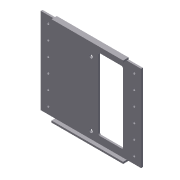
# Autodesk Inventor part: DriveTrain_MotorMount
Saved by Autodesk Inventor 2012 (Build 160160000, 160)
## iProperties
Created: 2012-01-08
Part Number: DriveTrain_MotorMount
Material: Aluminum-6061
Document SubType Name: Modeling
Designer: JesseK
Density: 2.71 g/cm^3
Mass: 222.88 g
Surface Area: 561.797 cm^2
Volume: 82.2435 cm^3
Author: JesseK
Autodesk Inventor part; units mm, degrees
ref_plane "YZ Plane" through (0, 0, 0) normal (1, 0, 0) x (0, 1, 0)
ref_plane "XZ Plane" through (0, 0, 0) normal (0, 1, 0) x (-1, 0, 0)
ref_plane "XY Plane" through (0, 0, 0) normal (0, 0, 1) x (1, 0, 0)
sketch "Sketch1" plane through (0, 0, 0) normal (0, 0, 1) x (1, 0, 0)
  line L0 (177.8, 0) -> (177.8, 152.4)
  line L1 (0, 152.4) -> (0, 0)
  line L2 (152.4, 152.4) -> (152.4, 155.575)
  line L3 (152.4, 155.575) -> (25.4, 155.575)
  line L4 (25.4, 155.575) -> (25.4, 152.4)
  line L5 (0, 152.4) -> (25.4, 152.4)
  line L6 (152.4, 152.4) -> (177.8, 152.4)
  line L7 (152.4, 0) -> (152.4, -3.175)
  line L8 (152.4, -3.175) -> (25.4, -3.175)
  line L9 (25.4, -3.175) -> (25.4, 0)
  line L10 (0, 0) -> (25.4, 0)
  line L11 (152.4, 0) -> (177.8, 0)
  dimension "d0" = 152.4
  dimension "d1" = 177.8
  dimension "d18" = 25.4
  dimension "d19" = 25.4
  dimension "d20" = 3.175
  constraints: 24 end point, 5 collinear, 4 perpendicular, 2 parallel, 1 vertical
  measures "d0" distance of L1.start L1.end
  measures "d1" distance of L1.end L0.start
  measures "d18" distance between parallel lines of L1 L4
  measures "d19" distance between parallel lines of L0 L2
  measures "d20" distance of L2.start L2.end
extrude "Extrusion3" add sketch "Sketch1" along normal blind 3.175
sketch "Sketch2" plane through (0, 0, 3.175) normal (0, 0, 1) x (1, 0, 0)
  line L0 (0, 152.4) -> (25.4, 152.4) projected
  line L1 (0, 0) -> (0, 152.4) projected
  line L2 (25.4, 0) -> (0, 0) projected
  line L3 (177.8, 0) -> (152.4, 0) projected
  line L4 (152.4, 152.4) -> (177.8, 152.4) projected
  line L5 (25.4, 152.4) -> (25.4, 155.575) projected
  line L6 (12.7, 152.4) -> (12.7, 139.7) construction
  line L7 (12.7, 139.7) -> (12.7, 114.3) construction
  line L8 (12.7, 114.3) -> (12.7, 88.9) construction
  line L9 (12.7, 88.9) -> (12.7, 63.5) construction
  line L10 (12.7, 63.5) -> (12.7, 38.1) construction
  line L11 (12.7, 38.1) -> (12.7, 12.7) construction
  line L12 (12.7, 12.7) -> (12.7, 0) construction
  circle A0 centre (12.7, 139.7) radius 2.3813
  circle A1 centre (12.7, 114.3) radius 2.3813
  circle A2 centre (12.7, 88.9) radius 2.3813
  circle A3 centre (12.7, 63.5) radius 2.3813
  circle A4 centre (12.7, 38.1) radius 2.3813
  circle A5 centre (12.7, 12.7) radius 2.3813
  line L13 (165.1, 152.4) -> (165.1, 139.7) construction
  line L14 (165.1, 139.7) -> (165.1, 114.3) construction
  line L15 (165.1, 114.3) -> (165.1, 88.9) construction
  line L16 (165.1, 88.9) -> (165.1, 63.5) construction
  line L17 (165.1, 63.5) -> (165.1, 38.1) construction
  line L18 (165.1, 38.1) -> (165.1, 12.7) construction
  line L19 (165.1, 12.7) -> (165.1, 0) construction
  circle A6 centre (165.1, 139.7) radius 2.3813
  circle A7 centre (165.1, 114.3) radius 2.3813
  circle A8 centre (165.1, 88.9) radius 2.3813
  circle A9 centre (165.1, 63.5) radius 2.3813
  circle A10 centre (165.1, 38.1) radius 2.3813
  circle A11 centre (165.1, 12.7) radius 2.3813
  dimension "d26" = 12.7
  dimension "d27" = 25.4
  dimension "d28" = 4.7625
  dimension "d29" = 12.7
  dimension "d30" = 25.4
  dimension "d31" = 4.7625
  constraints: 28 end point, 18 collinear, 12 centre point, 12 coincident, 10 equal radius, 4 midpoint, 3 parallel
  measures "d26" distance of L6.start L6.end
  measures "d27" distance of L6.end L7.end
  measures "d28" diameter of A2
  measures "d29" distance of L13.start L13.end
  measures "d30" distance of L13.end L14.end
  measures "d31" diameter of A6
extrude "Extrusion4" cut sketch "Sketch2" against normal up to next
sketch "Sketch3" plane through (0, 0, 3.175) normal (0, 0, 1) x (1, 0, 0)
  line L0 (0, 0) -> (0, 152.4) projected
  line L1 (25.4, 0) -> (0, 0) projected
  circle A0 centre (88.9, 127) radius 3.175
  circle A1 centre (88.9, 12.7) radius 3.175
  dimension "d34" = 88.9
  dimension "d35" = 88.9
  dimension "d36" = 114.3
  dimension "d37" = 12.7
  dimension "d38" = 6.35
  dimension "d39" = 6.35
  constraints: 2 centre point
  measures "d34" distance from line of A0.centre L0
  measures "d35" distance from line of L0 A1.centre
  measures "d36" distance of A0.centre A1.centre
  measures "d37" distance from line of L1 A1.centre
  measures "d38" diameter of A0
  measures "d39" diameter of A1
extrude "Extrusion5" cut sketch "Sketch3" against normal up to next
sketch "Sketch4" plane through (0, 0, 3.175) normal (0, 0, 1) x (1, 0, 0)
  circle A0 centre (88.9, 127) radius 3.175 projected
  line L0 (177.8, 0) -> (152.4, 0) projected
  line L1 (177.8, 152.4) -> (177.8, 0) projected
  line L2 (152.4, 152.4) -> (177.8, 152.4) projected
  line L3 (104.775, 139.7) -> (142.875, 139.7)
  line L4 (146.05, 136.525) -> (146.05, 15.875)
  line L5 (142.875, 12.7) -> (104.775, 12.7)
  line L6 (101.6, 15.875) -> (101.6, 136.525)
  arc A1 (104.775, 139.7) -> (101.6, 136.525) centre (104.775, 136.525) ccw
  arc A2 (146.05, 136.525) -> (142.875, 139.7) centre (142.875, 136.525) ccw
  arc A3 (142.875, 12.7) -> (146.05, 15.875) centre (142.875, 15.875) ccw
  arc A4 (101.6, 15.875) -> (104.775, 12.7) centre (104.775, 15.875) ccw
  dimension "d42" = 12.7
  dimension "d43" = 31.75
  dimension "d44" = 12.7
  dimension "d45" = 12.7
  dimension "d46" = 3.175
  constraints: 8 end point, 8 point on circle, 8 tangent, 4 centre point, 3 equal radius, 2 parallel, 1 horizontal, 1 perpendicular
  measures "d42" distance from line of L6 A0.centre
  measures "d43" distance between parallel lines of L1 L4
  measures "d44" distance between parallel lines of L2 L3
  measures "d45" distance between parallel lines of L0 L5
  measures "d46" radius of A1
extrude "Extrusion6" cut sketch "Sketch4" against normal up to next contours L3 A2 L4 A3 L5 A4 L6 A1
sketch "Sketch5" plane through (0, 0, 3.175) normal (0, 0, 1) x (1, 0, 0)
  line L0 (25.4, 155.575) -> (152.4, 155.575)
  line L1 (152.4, 155.575) -> (152.4, 152.4)
  line L2 (152.4, 152.4) -> (25.4, 152.4)
  line L3 (25.4, 152.4) -> (25.4, 155.575)
  line L4 (25.4, -3.175) -> (152.4, -3.175)
  line L5 (152.4, -3.175) -> (152.4, 0)
  line L6 (152.4, 0) -> (25.4, 0)
  line L7 (25.4, 0) -> (25.4, -3.175)
  constraints: 16 end point, 4 parallel, 2 horizontal, 2 perpendicular
extrude "Extrusion7" add sketch "Sketch5" along normal blind 6.35
body "Solid3"
